013 (Autodesk Fusion 360 design; units mm, degrees)
Autodesk Fusion 360 part; units mm, degrees
sketch "Esquisse1" plane through (0, 0, 0) normal (0, 0, 1) x (1, 0, 0)
  circle A0 centre (0, 0) radius 7.5
  dimension "d1" = 15
  constraint coincident A0.centre origin
  measures "d1" diameter of A0
extrude "Extrusion1" add sketch "Esquisse1" along normal blind 5
sketch "Esquisse2" plane through (0, 0, 0) normal (0, 1, 0) x (1, 0, 0)
sketch "Esquisse3" plane through (0, 0, 0) normal (0, 1, 0) x (1, 0, 0)
  line L0 (3, -3.5) -> (8.18, -4.4134)
  line L1 (8.18, -4.4134) -> (8.18, -0.5866)
  line L2 (8.18, -0.5866) -> (3, -1.5)
  line L3 (3, -1.5) -> (3, -3.5)
  line L4 (0, -1.75) -> (0, -22.5)
  dimension "d4" = 2
  dimension "d6" = 1.5
  dimension "d7" = 100
  dimension "d8" = 100
  dimension "d9" = 3
  constraint vertical L1
  constraint parallel L1 L3
  measures "d4" distance of L0.start L2.end
  measures "d6" vertical distance of L2.end origin
  measures "d7" angle of L2 L3
  measures "d8" angle of L0 L3
  measures "d9" distance of L3 L4
revolve "Révolution1" cut sketch "Esquisse3" angle 360 about axis through (0, 0, 1.75) along (0, 0, 1)
sketch "Esquisse4" plane through (0, 0, 5) normal (0, 0, 1) x (-1, 0, 0)
  circle A0 centre (0, 0) radius 7.5
  circle A1 centre (0, 0) radius 6
  dimension "d11" = 12
  constraint coincident A0.centre A1.centre
  measures "d11" diameter of A1
extrude "Extrusion2" add sketch "Esquisse4" along normal blind 8 contours A1
sketch "Esquisse5" plane through (0, 0, 13) normal (0, 0, 1) x (-1, 0, 0)
  circle A0 centre (0, 0) radius 6
  circle A1 centre (0, 0) radius 4.125
  dimension "d14" = 8.25
  constraint coincident A0.centre A1.centre
  measures "d14" diameter of A1
sketch "Esquisse6" plane through (0, 0, 13) normal (0, 0, 1) x (1, 0, 0)
extrude "Extrusion3" cut sketch "Esquisse5" against normal blind 7 contours A1
sketch "Esquisse7" plane through (0, 0, 0) normal (0, 1, 0) x (1, 0, 0)
  circle A0 centre (0, -10) radius 1.35
  line L0 (-6, -13) -> (6, -13)
  dimension "d17" = 2.7
  dimension "d18" = 3
  measures "d17" diameter of A0
  measures "d18" distance of A0.centre L0
extrude "Extrusion4" cut sketch "Esquisse7" along normal blind 15.5
